threadedBottomRod_v1 (Autodesk Fusion 360 design; units mm, degrees)
Autodesk Fusion 360 part; units mm, degrees
sketch "Sketch1" plane through (0, 0, 0) normal (0, 0, 1) x (1, 0, 0)
  circle A0 centre (0, 0) radius 3.175
  dimension "d1" = 6.35
  constraint coincident A0.centre origin
  measures "d1" diameter of A0
extrude "Extrude1" add sketch "Sketch1" along normal blind 38.1
thread "Thread1" "ANSI Unified Screw Threads 0.25 1/4-20 UNC 3A" major diameter 6.2484 minor diameter 4.8387 pitch 1.27 angle 60 resizes the face on face at (3.1711, -0.1583, 25.4) from (0, 0, 25.4) to (0, 0, 38.1)
chamfer "Chamfer1" distance 0.254 angle 45 1 edges at (-2.9128, -1.1298, 38.1)
sketch "Sketch2" plane through (0, 0, 0) normal (0, 0, -1) x (1, 0, 0)
  circle A0 centre (0, 0) radius 3.1242
  constraint coincident A0.centre origin
hole "Hole1" at (0, 0, 0) direction (0, 0, 1) diameter 1.271 depth 6.35 tip angle 118
thread "Thread2" "ANSI Metric M Profile 1.6 M1.6x0.35 6H"
